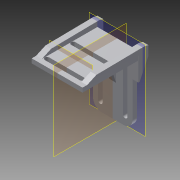
# Autodesk Inventor part: gimbal_pitch_brushless
Saved by Autodesk Inventor 2015 SP1 (Build 190203100, 203)
## iProperties
Created: 2015-08-06
Part Number: gimbal_pitch_brushless
Material: ABS Plastic
Document SubType Name: Modeling
Designer: Alexandre Cherpillod
Density: 1.06 g/cm^3
Appearance: Smooth - White
Mass: 2.62665 g
Surface Area: 30.5584 cm^2
Volume: 2.47797 cm^3
Author: Alexandre Cherpillod
Autodesk Inventor part; units mm, degrees
ref_plane "XY Plane" through (0, 0, 0) normal (0, 0, 1) x (1, 0, 0)
sketch "Sketch1" plane through (0, 0, 0) normal (0, 1, 0) x (-1, 0, 0)
  line L0 (-9, 20) -> (9, 20)
  line L1 (9, 20) -> (9, -10.6569)
  line L2 (9, -10.6569) -> (-9, -10.6569)
  line L3 (-9, -10.6569) -> (-9, 20)
  line L4 (-9, 20) -> (9, -10.6569) construction
  line L5 (9, 20) -> (-9, -10.6569) construction
  line L6 (0, -28.0453) -> (0, 28.0076) construction
  line L7 (-14.8076, 0) -> (25.8453, 0) construction
  line L8 (0, 0) -> (20.0378, -20.0378) construction
  line L9 (5.6569, -7.6569) -> (5.6569, 16.6569) construction
  line L10 (6.6569, -6.6569) -> (6.6569, 15.6569)
  line L11 (4.6569, 15.6569) -> (4.6569, -6.6569)
  arc A0 (4.6569, -6.6569) -> (6.6569, -6.6569) centre (5.6569, -6.6569) ccw
  arc A1 (6.6569, 15.6569) -> (4.6569, 15.6569) centre (5.6569, 15.6569) ccw
  line L12 (0, 0) -> (13.8345, 13.8345) construction
  line L13 (-5.6569, -7.6569) -> (-5.6569, 16.6569) construction
  line L14 (-6.6569, -6.6569) -> (-6.6569, 15.6569)
  line L15 (-4.6569, 15.6569) -> (-4.6569, -6.6569)
  arc A2 (-6.6569, -6.6569) -> (-4.6569, -6.6569) centre (-5.6569, -6.6569) ccw
  arc A3 (-4.6569, 15.6569) -> (-6.6569, 15.6569) centre (-5.6569, 15.6569) ccw
  point P0 (0, 4.6716)
  point P1 (0, 4.6716)
  point P2 (5.6569, -5.6569)
  point P3 (5.6569, 4.5)
  point P4 (5.6569, 5.6569)
  point P5 (-5.6569, -5.6569)
  point P6 (-5.6569, 4.5)
  point P7 (-5.6569, 5.6569)
  dimension "d34" = 18
  dimension "d35" = 45
  dimension "d36" = 8
  dimension "d37" = 2
  dimension "d38" = 1
  dimension "d40" = 45
  dimension "d41" = 10
  dimension "d42" = 4
  dimension "d43" = 20
  constraints: 32 end point, 13 point on line, 12 point on circle, 11 symmetric about line, 4 centre point, 4 midpoint, 4 tangent, 3 parallel, 1 horizontal, 1 perpendicular, 1 vertical, 2 other
  measures "d34" distance of L1.end L2.end
  measures "d35" angle of L6 L8
  measures "d36" distance of L8.start point (5.657, -5.657)
  measures "d37" diameter of A1
  measures "d38" distance of A0.centre point (5.657, -5.657)
  measures "d40" angle of L6 L12
  measures "d41" distance of A1.centre point (5.657, 5.657)
  measures "d42" distance from line of L2 A0.centre
  measures "d43" distance from line of L0 L8.start
extrude "Extrusion1" add sketch "Sketch1" against normal blind 2
sketch "Sketch5" plane through (-9, 0, 20) normal (0, 0, 1) x (1, 0, 0)
  line L0 (-2.5982, 0) -> (20.5467, 0)
  line L1 (20.5467, 0) -> (20.5467, -27.3268)
  line L2 (20.5467, -27.3268) -> (-2.5982, -27.3268)
  line L3 (-2.5982, -27.3268) -> (-2.5982, 0)
  line L4 (18, 0) -> (18, -2) construction
  line L5 (0, 0) -> (0, -2) projected
  line L6 (1, -24) -> (17, -24) construction
  line L7 (1, -25) -> (17, -25)
  line L8 (17, -23) -> (1, -23)
  arc A0 (1, -23) -> (1, -25) centre (1, -24) ccw
  arc A1 (17, -25) -> (17, -23) centre (17, -24) ccw
  line L9 (1, -12) -> (17, -12) construction
  line L10 (1, -13) -> (17, -13)
  line L11 (17, -11) -> (1, -11)
  arc A2 (1, -11) -> (1, -13) centre (1, -12) ccw
  arc A3 (17, -13) -> (17, -11) centre (17, -12) ccw
  line L12 (0, -2) -> (18, -2) projected
  point P0 (9, 0)
  point P1 (9, -24)
  point P2 (9, -12)
  dimension "d56" = 2
  dimension "d57" = 2
  dimension "d58" = 12
  dimension "d59" = 8
  dimension "d62" = 10
  constraints: 24 end point, 8 point on circle, 8 tangent, 6 parallel, 4 centre point, 2 horizontal, 2 midpoint, 1 perpendicular
  measures "d56" diameter of A1
  measures "d57" diameter of A3
  measures "d58" distance between parallel lines of L6 L9
  measures "d59" distance of L9.end point (9, -12)
  measures "d62" distance from line of L12 point (9, -12)
extrude "Extrusion5" add sketch "Sketch5" against normal blind 2
ref_plane "Work Plane1" through (-8, -18, 20) normal (0, -1, 0) x (1, 0, 0)
fillet "Fillet2" radius 4 2 edges at (-9, -1, -10.6569) (9, -1, -10.6569)
sketch "Sketch6" plane through (0, 0, 0) normal (1, 0, 0) x (0, 1, 0)
  line L0 (-2, 4.2697) -> (-6.6287, 18)
  line L1 (-6.6287, 18) -> (-2, 18)
  line L2 (-2, 18) -> (-2, -6.6569) projected
  line L3 (-2, 18) -> (-2, 4.2697)
  point P0 (0, 0)
  constraints: 6 end point, 1 collinear, 1 perpendicular
extrude "Extrusion6" add sketch "Sketch6" along normal mid plane 3
sketch "Sketch7" plane through (-9, -2, 18) normal (-1, 0, 0) x (0, 0, 1)
  line L0 (-8.6385, 0.6553) -> (-0.5065, 4.6311)
  line L1 (-0.5065, 4.6311) -> (3.8294, 4.6311)
  line L2 (3.8294, 4.6311) -> (4.27, 2.7989)
  line L3 (4.27, 2.7989) -> (3.937, -19.0711)
  line L4 (3.937, -19.0711) -> (2, -23.3264)
  line L5 (-8.6385, 0.6553) -> (-8.6385, 0)
  line L6 (2, 0) -> (2, -23.3264)
  line L7 (2, 0) -> (-8.6385, 0)
  line L8 (0, 0) -> (-24.6569, 0) projected
  point P0 (-18, 2)
  point P1 (2, 2)
  constraints: 16 end point, 1 collinear, 1 point on line, 1 vertical
extrude "Extrusion7" add sketch "Sketch7" along normal up to surface (2.5982 mm away)
mirror "Mirror1" about plane through (0, 0, 0) normal (1, 0, 0) of "Extrusion7"
body "Solid1"
